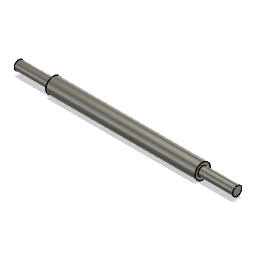
main (Autodesk Fusion 360 archive; units mm, degrees)
design "watch_band_pin"
Autodesk Fusion 360 part; units mm, degrees
sketch "Sketch1" plane through (0, 0, 0) normal (0, 1, 0) x (1, 0, 0)
  line L0 (0, 0) -> (10.75, 0)
  line L1 (0, 0) -> (0, 0.75) construction
  line L2 (10.75, 0) -> (10.75, 0.45)
  line L3 (10.75, 0.45) -> (7.35, 0.45)
  line L4 (7.35, 0.45) -> (7.35, 0.75)
  line L5 (0, 0.75) -> (7.35, 0.75)
  line L6 (-10.75, 0) -> (-10.75, 0.45)
  line L7 (-10.75, 0.45) -> (-7.35, 0.45)
  line L8 (-7.35, 0.45) -> (-7.35, 0.75)
  line L9 (0, 0.75) -> (-7.35, 0.75)
  line L10 (-10.75, 0) -> (0, 0)
  dimension "d1" = 0.75
  dimension "d2" = 10.75
  dimension "d3" = 0.45
  dimension "d4" = 3.4
  constraint coincident L0.start L1.start
  constraint horizontal L0
  constraint perpendicular L0 L1
  constraint perpendicular L0 L2
  constraint perpendicular L2 L3
  constraint perpendicular L3 L4
  constraint coincident L4 L5.end
  constraint perpendicular L4 L5
  constraint symmetric L0.end L1 L6.start
  constraint symmetric L5.start L1 L9.start
  constraint symmetric L1 L2.end L6.end
  constraint symmetric L1 L3.end L7.end
  constraint symmetric L1 L4.end L8.end
  measures "d1" distance of L0.start L1.end
  measures "d2" distance of L0.start L0.end
  measures "d3" distance of L0.end L2.end
  measures "d4" distance of L2.end L3.end
revolve "Revolve1" add sketch "Sketch1" angle 360 about axis through (0, 0, 0) along (1, 0, 0)
equation "d1 = ( 1.5 / 2 ) * 1 mm"
equation "d2 = ( 21.5 / 2 ) * 1 mm"
equation "d3 = ( 0.9 / 2 ) * 1 mm"

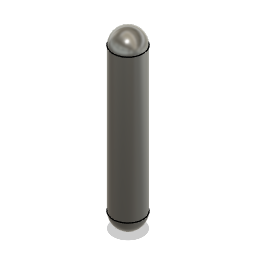
design "tag"
Autodesk Fusion 360 part; units mm, degrees
sketch "Sketch1" plane through (0, 0, 0) normal (0, 0, 1) x (1, 0, 0)
  line L0 (0, 0) -> (0, 6.25) construction
  line L1 (0, 0) -> (1.075, 0) construction
  line L2 (-1.075, 5.175) -> (-1.075, -5.175) construction
  arc A0 (0, -6.25) -> (1.075, -5.175) centre (0, -5.175) ccw
  line L3 (1.075, -5.175) -> (1.075, 5.175)
  arc A1 (1.075, 5.175) -> (0, 6.25) centre (0, 5.175) ccw
  line L4 (0, 6.25) -> (0, -6.25)
  arc A2 (0, 6.25) -> (-1.075, 5.175) centre (0, 5.175) ccw construction
  arc A3 (-1.075, -5.175) -> (0, -6.25) centre (0, -5.175) ccw construction
  dimension "d1" = 6.25
  dimension "d2" = 1.075
  constraint coincident L0.start L1.start
  constraint vertical L0
  constraint perpendicular L0 L1
  constraint symmetric L0.end L1 A0.start
  constraint tangent L2 A0
  constraint tangent A0 L3
  constraint parallel L2 L3
  constraint tangent L3 A1
  constraint tangent L2 A1
  constraint midpoint A0 L4.end
  constraint coincident A0.start L4.end
  constraint concentric A1 A2
  constraint concentric A0 A3
  measures "d1" distance of L0.start L0.end
  measures "d2" distance of L0.start L1.end
revolve "Revolve1" add sketch "Sketch1" angle 360 about axis through (0, 6.25, 0) along (0, -1, 0)
equation "d1 = ( 12.5 / 2 ) * 1 mm"
equation "d2 = ( 2.15 / 2 ) * 1 mm"
